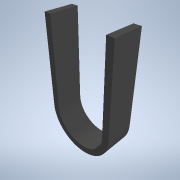
# Autodesk Inventor part: Belt_A
Saved by Autodesk Inventor 2020 (Build 240168000, 168)
## iProperties
Created: 2020-03-07
Part Number: Belt_A
Material: Rubber
Document SubType Name: Modeling
Designer: 10300812
Density: 0.93 g/cm^3
Appearance: Rubber - Black
Author: 10300812
Autodesk Inventor part; units mm, degrees
ref_plane "YZ Plane" through (0, 0, 0) normal (1, 0, 0) x (0, 1, 0)
ref_plane "XZ Plane" through (0, 0, 0) normal (0, 1, 0) x (-1, 0, 0)
ref_plane "XY Plane" through (0, 0, 0) normal (0, 0, 1) x (1, 0, 0)
sketch "Sketch1" plane through (0, 0, 0) normal (0, 0, 1) x (1, 0, 0)
  arc A0 (-5.6377, -2.1951) -> (5.6377, -2.1951) centre (0, 0) ccw
  arc A1 (-7.0355, -2.7394) -> (7.0355, -2.7394) centre (0, 0) ccw
  circle A2 centre (-20.5, 52.65) radius 3 projected
  circle A3 centre (20.5, 52.65) radius 3 projected
  arc A4 (-20.5, 58.7) -> (-26.1377, 50.4549) centre (-20.5, 52.65) ccw
  arc A5 (26.1377, 50.4549) -> (20.5, 58.7) centre (20.5, 52.65) ccw
  arc A6 (-20.5, 60.2) -> (-27.5355, 49.9106) centre (-20.5, 52.65) ccw
  arc A7 (27.5355, 49.9106) -> (20.5, 60.2) centre (20.5, 52.65) ccw
  line L0 (-7.0355, -2.7394) -> (-27.5355, 49.9106)
  line L1 (-26.1377, 50.4549) -> (-5.6377, -2.1951)
  line L2 (7.0355, -2.7394) -> (27.5355, 49.9106)
  line L3 (5.6377, -2.1951) -> (26.1377, 50.4549)
  line L4 (-20.5, 60.2) -> (20.5, 60.2)
  line L5 (20.5, 58.7) -> (-20.5, 58.7)
  dimension "d0" = 12.1
  dimension "d4" = 12.1
  dimension "d5" = 12.1
  dimension "d6" = 1.5
  dimension "d7" = 1.5
  constraints: 12 end point, 12 point on circle, 8 tangent, 6 centre point, 3 coincident, 3 parallel, 1 horizontal alignment
  measures "d0" diameter of A0
  measures "d4" diameter of A4
  measures "d5" diameter of A5
  measures "d6" radial gap between concentric circles of A4 A6
  measures "d7" radial gap between concentric circles of A5 A7
extrude "Extrusion1" add sketch "Sketch1" along normal blind 6 contours L0 A6 L4 A7 L2 A1
body "Solid1"
